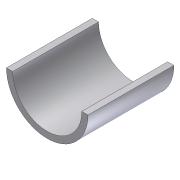
# Autodesk Inventor part: FE-00013-01
Saved by Autodesk Inventor 2012 (Build 160160000, 160)
## iProperties
Created: 2008-05-28
Part Number: FE-00013-01
Description: Rail Cradle
Document SubType Name: Modeling
Designer: narosenberg
Density: 1 g/cm^3
Mass: 13.1009 g
Surface Area: 80.0414 cm^2
Volume: 13.1009 cm^3
Material: Default
Author: narosenberg
Autodesk Inventor part; units mm, degrees
ref_plane "YZ Plane" through (0, 0, 0) normal (1, 0, 0) x (0, 1, 0)
ref_plane "XZ Plane" through (0, 0, 0) normal (0, 1, 0) x (-1, 0, 0)
ref_plane "XY Plane" through (0, 0, 0) normal (0, 0, 1) x (1, 0, 0)
sketch "Sketch1" plane through (0, 0, 0) normal (0, 0, 1) x (1, 0, 0)
  arc A0 (-29.2796, 12.7254) -> (11.6144, 12.7254) centre (-8.8326, 12.7254) ccw
  arc A1 (-32.9626, 12.7254) -> (15.2974, 12.7254) centre (-8.8326, 12.7254) ccw
  line L0 (-8.8326, 12.7254) -> (-8.8326, -11.4046)
  line L1 (-32.9626, 12.7254) -> (15.2974, 12.7254)
  dimension "d0" = 40.894
  dimension "d1" = 48.26
  dimension "d4" = 24.13
  constraints: 5 point on circle, 4 end point, 2 centre point, 2 point on line, 1 coincident, 1 perpendicular
  measures "d0" diameter of A0
  measures "d1" diameter of A1
  measures "d4" distance from line of L0.end L1
extrude "Extrusion1" add sketch "Sketch1" along normal blind 50.8 contours A0 L0 A1 L1 | A0 L1 A1 L0
body "Solid1"
